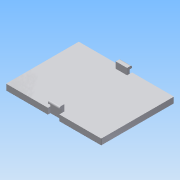
# Autodesk Inventor part: D2MG крышка
Saved by Autodesk Inventor 2015 SP1 (Build 190203100, 203)
## iProperties
Created: 2017-11-06
Part Number: D2MG крышка
Material: Типовые
Document SubType Name: Modeling
Designer: Влад
Density: 1 g/cm^3
Appearance: Белый пластик
Author: Влад
Autodesk Inventor part; units mm, degrees
ref_plane "YZ Plane" through (0, 0, 0) normal (1, 0, 0) x (0, 1, 0)
ref_plane "XZ Plane" through (0, 0, 0) normal (0, 1, 0) x (-1, 0, 0)
ref_plane "XY Plane" through (0, 0, 0) normal (0, 0, 1) x (1, 0, 0)
sketch "Эскиз1" plane through (0, 0, 0) normal (0, 0, 1) x (1, 0, 0)
  line L0 (-21, 16.05) -> (21, 16.05)
  line L1 (21, 16.05) -> (21, -16.05)
  line L2 (21, -16.05) -> (-21, -16.05)
  line L3 (-21, -16.05) -> (-21, 16.05)
  line L4 (-21, 16.05) -> (21, -16.05) construction
  line L5 (21, 16.05) -> (-21, -16.05) construction
  point P0 (0, 0)
  point P1 (0, 0)
  dimension "d0" = 42
  dimension "d1" = 32.1
  constraints: 12 end point, 2 parallel, 1 coincident, 1 horizontal, 1 midpoint, 1 perpendicular
  measures "d0" distance of L1.end L2.end
  measures "d1" distance of L0.end L1.end
extrude "Выдавливание1" add sketch "Эскиз1" along normal blind 2.7
sketch "Эскиз3" plane through (0, 0, 2.7) normal (0, 0, 1) x (1, 0, 0)
  line L0 (-2.5, 16.05) -> (2.5, 16.05)
  line L1 (2.5, 16.05) -> (2.5, 15.05)
  line L2 (2.5, 15.05) -> (-2.5, 15.05)
  line L3 (-2.5, 15.05) -> (-2.5, 16.05)
  line L4 (-2.5, -15.05) -> (2.5, -15.05)
  line L5 (2.5, -15.05) -> (2.5, -16.05)
  line L6 (2.5, -16.05) -> (-2.5, -16.05)
  line L7 (-2.5, -16.05) -> (-2.5, -15.05)
  line L8 (-21, -16.05) -> (21, -16.05) projected
  line L9 (21, 16.05) -> (-21, 16.05) projected
  line L10 (-21, 16.05) -> (-21, -16.05) projected
  line L11 (21, -16.05) -> (21, 16.05) projected
  point P0 (0, 0)
  point P1 (0, -16.05)
  point P2 (0, 16.05)
  dimension "d10" = 5
  dimension "d11" = 1
  dimension "d12" = 5
  dimension "d13" = 1
  dimension "d14" = 18.5
  dimension "d15" = 18.5
  dimension "d16" = 18.5
  dimension "d17" = 18.5
  constraints: 16 end point, 4 midpoint, 4 parallel, 2 horizontal, 2 perpendicular
  measures "d10" distance of L1.end L2.end
  measures "d11" distance of L0.end L1.end
  measures "d12" distance of L5.end L6.end
  measures "d13" distance of L4.end L5.end
  measures "d14" distance between parallel lines of L10 L3
  measures "d15" distance between parallel lines of L10 L7
  measures "d16" distance between parallel lines of L11 L5
  measures "d17" distance between parallel lines of L11 L1
extrude "Выдавливание3" cut sketch "Эскиз3" against normal blind 2.7 contours L0 L1 L2 L3 | L7 L4 L5 L6
sketch "Эскиз4" plane through (2.5, -16.05, 2.7) normal (-1, 0, 0) x (0, 0, 1)
  line L0 (0, 1) -> (0, 2.2)
  line L1 (0, 31.1) -> (0, 1) projected
  line L2 (0, 2.2) -> (2.8, 2.2)
  line L3 (2.8, 2.2) -> (2.8, 0.75)
  line L4 (1.7, 0) -> (2.05, 0)
  line L5 (1.7, 1) -> (1.7, 0)
  line L6 (0, 1) -> (1.7, 1)
  arc A0 (2.05, 0) -> (2.8, 0.75) centre (2.05, 0.75) ccw
  line L7 (7.4622, 16.05) -> (-10.2313, 16.05) construction
  line L8 (-2.7, 32.1) -> (0, 32.1) construction
  line L9 (0, 31.1) -> (0, 29.9)
  line L10 (0, 29.9) -> (2.8, 29.9)
  line L11 (2.8, 29.9) -> (2.8, 31.35)
  line L12 (1.7, 32.1) -> (2.05, 32.1)
  line L13 (1.7, 31.1) -> (1.7, 32.1)
  line L14 (0, 31.1) -> (1.7, 31.1)
  arc A1 (2.8, 31.35) -> (2.05, 32.1) centre (2.05, 31.35) ccw
  point P0 (-2.7, 16.05)
  point P1 (2.8, 0)
  point P2 (0, 0)
  point P3 (2.8, 32.1)
  dimension "d20" = 1.2
  dimension "d21" = 2.8
  dimension "d22" = 1.1
  dimension "d23" = 0.75
  dimension "d24" = 16.05
  constraints: 26 end point, 8 symmetric about line, 5 point on line, 4 point on circle, 3 horizontal, 2 centre point, 2 perpendicular, 2 tangent, 1 vertical, 1 other
  measures "d20" distance of L0.start L0.end
  measures "d21" distance of L0.end L2.end
  measures "d22" distance of L4.start point (2.8, 0)
  measures "d23" radius of A0
  measures "d24" distance between parallel lines of L8 L7
extrude "Выдавливание4" add sketch "Эскиз4" along normal blind 5
sketch "Эскиз5" plane through (0, 0, 0) normal (0, 0, -1) x (-1, 0, 0)
  line L0 (20, -15.05) -> (-20, -15.05)
  line L1 (-20, -15.05) -> (-20, 15.05)
  line L2 (-20, 15.05) -> (20, 15.05)
  line L3 (20, 15.05) -> (20, -15.05)
  line L4 (2.5, -16.05) -> (21, -16.05) projected
  line L5 (21, -16.05) -> (21, 16.05) projected
  point P0 (0, 0)
  dimension "d27" = 40
  dimension "d28" = 30.1
  dimension "d29" = 1
  dimension "d30" = 1
  constraints: 8 end point, 2 parallel, 1 horizontal, 1 perpendicular
  measures "d27" distance of L1.end L2.end
  measures "d28" distance of L0.end L1.end
  measures "d29" distance between parallel lines of L4 L0
  measures "d30" distance between parallel lines of L5 L3
extrude "Выдавливание5" cut sketch "Эскиз5" against normal blind 0.2
fillet "Сопряжение1" radius 0.2 14 edges at (-21, 0, 0) (-11.75, -16.05, 0) (11.75, -16.05, 0) (21, 0, 0) (11.75, 16.05, 0) (-11.75, 16.05, 0) (-2.5, 15.55, 0) (2.5, 15.55, 0) (-2.5, -15.55, 0) (2.5, -15.55, 0) (-21, 16.05, 1.35) (-21, -16.05, 1.35) (21, 16.05, 1.35) (21, -16.05, 1.35)
fillet "Сопряжение2" radius 0.05 12 edges at (2.5586, 15.05, 0.0586) (11.35, 15.05, 0) (20, 0, 0) (2.5586, -15.05, 0.0586) (11.35, -15.05, 0) (0, -15.05, 0.2) (-11.35, -15.05, 0) (-2.5586, -15.05, 0.0586) (-20, 0, 0) (-2.5586, 15.05, 0.0586) (-11.35, 15.05, 0) (0, 15.05, 0.2)
